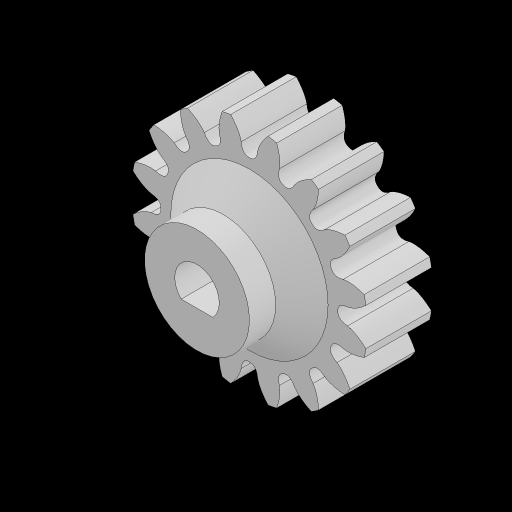
# Autodesk Inventor part: Motor Drive Gear V2
Saved by Autodesk Inventor 2023.2 (Build 272271030, 271C)
## iProperties
Created: 2023-11-17
Part Number: Motor Drive Gear V2
Material: Generic
Document SubType Name: Modeling
Designer: robpl
Density: 1 g/cm^3
Appearance: Default
Author: robpl
Autodesk Inventor part; units mm, degrees
ref_plane "YZ Plane" through (0, 0, 0) normal (1, 0, 0) x (0, 1, 0)
ref_plane "XZ Plane" through (0, 0, 0) normal (0, 1, 0) x (-1, 0, 0)
ref_plane "XY Plane" through (0, 0, 0) normal (0, 0, 1) x (1, 0, 0)
sketch "Sketch1" plane through (0, 0, 0) normal (0, 0, 1) x (1, 0, 0)
  spline S0 degree 3 poles (-1.4281, 8.886) (-1.3828, 8.8354) (-1.2923, 8.7343) (-1.1651, 8.5753) (-1.0451, 8.4108) (-0.934, 8.2402) (-0.8328, 8.0634) (-0.7586, 7.9107) (-0.7067, 7.7853) (-0.6725, 7.6895) (-0.6427, 7.592) (-0.6311, 7.5251) (-0.6253, 7.4917) knots 0 0 0 0 0.020354 0.040707 0.06106 0.081413 0.101765 0.122116 0.132293 0.142469 0.152645 0.162815 0.162815 0.162815 0.162815
  spline S1 degree 3 poles (-0.6253, 7.4917) (-0.6216, 7.4461) (-0.616, 7.3776) (-0.6009, 7.2873) (-0.5848, 7.2206) (-0.5652, 7.1547) (-0.54, 7.0908) (-0.5101, 7.029) (-0.4741, 6.9704) (-0.4319, 6.9161) (-0.3833, 6.8675) (-0.3287, 6.8255) (-0.269, 6.7913) (-0.2047, 6.7667) (-0.1373, 6.7519) (-0.0686, 6.7491) (0, 6.7504) (0.0686, 6.7491) (0.1373, 6.7519) (0.2047, 6.7667) (0.269, 6.7913) (0.3287, 6.8255) (0.3833, 6.8675) (0.4319, 6.9161) (0.4741, 6.9704) (0.5101, 7.029) (0.54, 7.0908) (0.5652, 7.1547) (0.5848, 7.2206) (0.6009, 7.2873) (0.616, 7.3776) (0.6216, 7.4461) (0.6253, 7.4917) knots 0 0 0 0 0.013722 0.020586 0.027448 0.034312 0.041173 0.048034 0.054897 0.061759 0.068618 0.075477 0.082338 0.089199 0.096059 0.102917 0.10978 0.116643 0.123501 0.130362 0.137223 0.144084 0.150942 0.157802 0.164663 0.171526 0.178387 0.185249 0.192112 0.198975 0.205838 0.219561 0.219561 0.219561 0.219561
  spline S2 degree 3 poles (0.6253, 7.4917) (0.6311, 7.5251) (0.6427, 7.592) (0.6725, 7.6895) (0.7067, 7.7853) (0.7586, 7.9107) (0.8328, 8.0634) (0.934, 8.2402) (1.0451, 8.4108) (1.1651, 8.5753) (1.2923, 8.7343) (1.3828, 8.8354) (1.4281, 8.886) knots 0 0 0 0 0.01017 0.020346 0.030522 0.040699 0.06105 0.081402 0.101754 0.122108 0.142461 0.162815 0.162815 0.162815 0.162815
  circle A0 centre (0, 0) radius 6.75 construction
  circle A1 centre (0, 0) radius 7.5175 construction
  circle A2 centre (0, 0) radius 8 construction
  circle A3 centre (0, 0) radius 9
  point P0 (-1.2937, 8.7331)
  point P1 (-1.1663, 8.5744)
  point P2 (-1.0466, 8.4098)
  point P3 (-0.9356, 8.2391)
  point P4 (-0.8348, 8.0623)
  point P5 (-0.7462, 7.8791)
  point P6 (-0.7075, 7.785)
  point P7 (-0.6732, 7.6892)
  point P8 (-0.6448, 7.5915)
  point P9 (-0.6116, 7.3551)
  point P10 (-0.6001, 7.2875)
  point P11 (-0.5842, 7.2207)
  point P12 (-0.5642, 7.1551)
  point P13 (-0.5392, 7.0912)
  point P14 (-0.5091, 7.0295)
  point P15 (-0.4731, 6.9711)
  point P16 (-0.4308, 6.9171)
  point P17 (-0.3823, 6.8686)
  point P18 (-0.3279, 6.8268)
  point P19 (-0.2682, 6.7929)
  point P20 (-0.2042, 6.7683)
  point P21 (-0.1371, 6.7539)
  point P22 (-0.0686, 6.7498)
  point P23 (0, 6.75)
  point P24 (0.0686, 6.7498)
  point P25 (0.1371, 6.7539)
  point P26 (0.2042, 6.7683)
  point P27 (0.2682, 6.7929)
  point P28 (0.3279, 6.8268)
  point P29 (0.3823, 6.8686)
  point P30 (0.4308, 6.9171)
  point P31 (0.4731, 6.9711)
  point P32 (0.5091, 7.0295)
  point P33 (0.5392, 7.0912)
  point P34 (0.5642, 7.1551)
  point P35 (0.5842, 7.2207)
  point P36 (0.6001, 7.2875)
  point P37 (0.6116, 7.3551)
  point P38 (0.6448, 7.5915)
  point P39 (0.6732, 7.6892)
  point P40 (0.7075, 7.785)
  point P41 (0.7462, 7.8791)
  point P42 (0.8348, 8.0623)
  point P43 (0.9356, 8.2391)
  point P44 (1.0466, 8.4098)
  point P45 (1.1663, 8.5744)
  point P46 (1.2937, 8.7331)
  constraints: 4 centre point, 2 point on circle, 109 other
extrude "Extrusion1" add sketch "Sketch1" against normal blind 5
extrude "Extrusion2" cut sketch "Sketch1" against normal through all contours A3 S2 S1 S0 picked at (0.1465, 8.2466)
pattern_circular "Circular Pattern1" count 16 over 360 about axis through (0, 0, 0) along (0, 0, -1) of "Extrusion2"
sketch "Sketch2" plane through (0, 0, 0) normal (0, 0, 1) x (1, 0, 0)
  arc A0 (1.118, -1) -> (-1.118, -1) centre (0, 0) ccw
  line L0 (-1.118, -1) -> (1.118, -1)
  arc A1 (1.2042, -1.2) -> (-1.2042, -1.2) centre (0, 0) ccw
  line L1 (1.2042, -1.2) -> (-1.2042, -1.2)
  point P0 (0, 1.5)
  dimension "d7" = 3
  dimension "d8" = 2.5
  dimension "d9" = 0.2
  constraints: 5 point on circle, 4 end point, 2 centre point, 1 coincident, 1 horizontal, 1 other
  measures "d7" diameter of A0
  measures "d9" radial gap between concentric circles of A0 A1
extrude "Extrusion3" cut sketch "Sketch2" against normal through all contours L0 A0 | L1 A1
sketch "Sketch3" plane through (0, 0, 0) normal (0, 0, 1) x (1, 0, 0)
  circle A0 centre (0, 0) radius 4
  arc A1 (1.2042, -1.2) -> (-1.2042, -1.2) centre (0, 0) ccw projected
  line L0 (1.2042, -1.2) -> (-1.2042, -1.2) projected
  arc A2 (-4.7199, 7.6631) -> (-5.2735, 7.2931) centre (0, 0) ccw projected
  arc A3 (-7.2931, 5.2735) -> (-7.6631, 4.7199) centre (0, 0) ccw projected
  arc A4 (-8.7561, 2.0812) -> (-8.886, 1.4281) centre (0, 0) ccw projected
  arc A5 (-8.886, -1.4281) -> (-8.7561, -2.0812) centre (0, 0) ccw projected
  arc A6 (-7.6631, -4.7199) -> (-7.2931, -5.2735) centre (0, 0) ccw projected
  arc A7 (-5.2735, -7.2931) -> (-4.7199, -7.6631) centre (0, 0) ccw projected
  arc A8 (-2.0812, -8.7561) -> (-1.4281, -8.886) centre (0, 0) ccw projected
  arc A9 (1.4281, -8.886) -> (2.0812, -8.7561) centre (0, 0) ccw projected
  arc A10 (4.7199, -7.6631) -> (5.2735, -7.2931) centre (0, 0) ccw projected
  arc A11 (7.2931, -5.2735) -> (7.6631, -4.7199) centre (0, 0) ccw projected
  arc A12 (8.7561, -2.0812) -> (8.886, -1.4281) centre (0, 0) ccw projected
  arc A13 (8.886, 1.4281) -> (8.7561, 2.0812) centre (0, 0) ccw projected
  arc A14 (7.6631, 4.7199) -> (7.2931, 5.2735) centre (0, 0) ccw projected
  arc A15 (5.2735, 7.2931) -> (4.7199, 7.6631) centre (0, 0) ccw projected
  arc A16 (2.0812, 8.7561) -> (1.4281, 8.886) centre (0, 0) ccw projected
  arc A17 (-1.4281, 8.886) -> (-2.0812, 8.7561) centre (0, 0) ccw projected
  point P0 (-2.2893, 7.1607)
  point P1 (-3.4446, 6.6821)
  point P2 (-4.8553, 5.7396)
  point P3 (-5.7396, 4.8553)
  point P4 (-6.6821, 3.4446)
  point P5 (-7.1607, 2.2893)
  point P6 (-7.4917, 0.6253)
  point P7 (-7.4917, -0.6253)
  point P8 (-7.1607, -2.2893)
  point P9 (-6.6821, -3.4446)
  point P10 (-5.7396, -4.8553)
  point P11 (-4.8553, -5.7396)
  point P12 (-3.4446, -6.6821)
  point P13 (-2.2893, -7.1607)
  point P14 (-0.6253, -7.4917)
  point P15 (0.6253, -7.4917)
  point P16 (2.2893, -7.1607)
  point P17 (3.4446, -6.6821)
  point P18 (4.8553, -5.7396)
  point P19 (5.7396, -4.8553)
  point P20 (6.6821, -3.4446)
  point P21 (7.1607, -2.2893)
  point P22 (7.4917, -0.6253)
  point P23 (7.4917, 0.6253)
  point P24 (7.1607, 2.2893)
  point P25 (6.6821, 3.4446)
  point P26 (5.7396, 4.8553)
  point P27 (4.8553, 5.7396)
  point P28 (3.4446, 6.6821)
  point P29 (2.2893, 7.1607)
  point P30 (0.6253, 7.4917)
  point P31 (-0.6253, 7.4917)
  dimension "d12" = 8
  constraints: 2 horizontal alignment, 2 vertical alignment, 1 centre point, 1 coincident, 44 other
  measures "d12" diameter of A0
extrude "Extrusion4" add sketch "Sketch3" along normal blind 4
chamfer "Chamfer1" distance 2 angle 45 1 edges at (-4, 0, 0)
equation "\"Module\" = 1"
equation "\"PressureAngle\" = 20deg"
equation "\"UnitProfileClearance\" = 0.25"
equation "\"UnitRoundRadius\" = 0.35"
equation "\"HeadDiameter\" = 18"
equation "\"RootDiameter\" = 13.5"
equation "\"BaseDiameter\" = 15.03508"
equation "\"PitchDiameter\" = 16"
equation "\"HelixAngle\" = 0"
equation "\"UnitCorrection\" = 0"
equation "\"UnitAddendumModification\" = 0"
equation "\"CircularPitch\" = 3.141593"
equation "\"UnitBacklashShift\" = 0"
equation "\"TotalToolShift\" = 0"
equation "\"IsInternal\" = 0"
body "Solid1"
